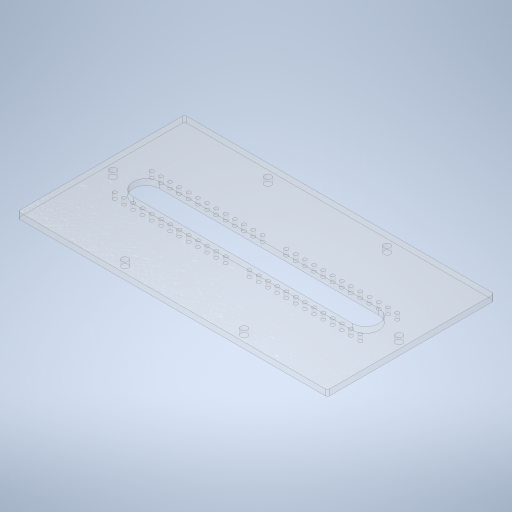
# Autodesk Inventor part: BT001_trajan20_21
Saved by Autodesk Inventor 2023 (Build 270158000, 158)
## iProperties
Company: HTBLA Kaindorf
RuleStatus: InUse
Created: 2022-08-03
Part Number: BT001_trajan20_21
Project: Zeichenmaschine_v2
Material: Acryl
Description: Platte Stepper Motoren
Document SubType Name: Modeling
Designer: trajan20
Density: 1.188 g/cm^3
Appearance: Transparent - farblos
Mass: 210.497 g
Surface Area: 764.437 cm^2
Volume: 177.186 cm^3
AfterDocNew0: iProperties-Editor_aufrufen
Author: jan
Keywords: 2021
Autodesk Inventor part; units mm, degrees
ref_plane "YZ Plane" through (0, 0, 0) normal (1, 0, 0) x (0, 1, 0)
ref_plane "XZ Plane" through (0, 0, 0) normal (0, 1, 0) x (-1, 0, 0)
ref_plane "XY Plane" through (0, 0, 0) normal (0, 0, 1) x (1, 0, 0)
derived "BT000_trajan20_22_Zeichenmaschine_neu_Masterskizze.ipt"
sketch "Skizze3" plane through (0, 0, 0) normal (0, 0, 1) x (1, 0, 0)
  line L0 (0, 0) -> (-140, 0)
  line L1 (-140, 0) -> (-140, 130)
  line L2 (-140, 260) -> (0, 260)
  line L3 (0, 260) -> (0, 0)
  line L4 (-140, 130) -> (-140, 260)
  line L5 (-70, 38) -> (-70, 222) construction
  line L6 (-81, 38) -> (-81, 222)
  line L7 (-59, 222) -> (-59, 38)
  arc A0 (-81, 38) -> (-59, 38) centre (-70, 38) ccw
  arc A1 (-59, 222) -> (-81, 222) centre (-70, 222) ccw
  circle A2 centre (-85.5, 27) radius 1.55
  circle A3 centre (-85.5, 58) radius 1.55
  circle A4 centre (-85.5, 34.75) radius 1.55
  circle A5 centre (-85.5, 42.5) radius 1.55
  line L8 (-85.5, 27) -> (-85.5, 242) construction
  circle A6 centre (-85.5, 50.25) radius 1.55
  line L9 (-88, 61.875) -> (-83, 61.875) construction
  circle A7 centre (-85.5, 96.75) radius 1.55
  circle A8 centre (-85.5, 89) radius 1.55
  circle A9 centre (-85.5, 81.25) radius 1.55
  circle A10 centre (-85.5, 73.5) radius 1.55
  circle A11 centre (-85.5, 65.75) radius 1.55
  line L10 (-88, 100.625) -> (-83, 100.625) construction
  circle A12 centre (-85.5, 112.25) radius 1.55
  circle A13 centre (-85.5, 120) radius 1.55
  circle A14 centre (-85.5, 104.5) radius 1.55
  line L11 (-70, 130) -> (-102, 130) construction
  circle A15 centre (-85.5, 225.25) radius 1.55
  circle A16 centre (-85.5, 217.5) radius 1.55
  circle A17 centre (-85.5, 209.75) radius 1.55
  circle A18 centre (-85.5, 202) radius 1.55
  circle A19 centre (-85.5, 194.25) radius 1.55
  circle A20 centre (-85.5, 186.5) radius 1.55
  circle A21 centre (-85.5, 178.75) radius 1.55
  circle A22 centre (-85.5, 171) radius 1.55
  circle A23 centre (-85.5, 163.25) radius 1.55
  circle A24 centre (-85.5, 155.5) radius 1.55
  circle A25 centre (-85.5, 147.75) radius 1.55
  circle A26 centre (-85.5, 140) radius 1.55
  circle A27 centre (-54.5, 27) radius 1.55
  circle A28 centre (-54.5, 34.75) radius 1.55
  circle A29 centre (-54.5, 42.5) radius 1.55
  circle A30 centre (-54.5, 50.25) radius 1.55
  circle A31 centre (-54.5, 58) radius 1.55
  circle A32 centre (-54.5, 65.75) radius 1.55
  circle A33 centre (-54.5, 73.5) radius 1.55
  circle A34 centre (-54.5, 81.25) radius 1.55
  circle A35 centre (-54.5, 89) radius 1.55
  circle A36 centre (-54.5, 96.75) radius 1.55
  circle A37 centre (-54.5, 104.5) radius 1.55
  circle A38 centre (-54.5, 112.25) radius 1.55
  circle A39 centre (-54.5, 120) radius 1.55
  circle A40 centre (-54.5, 140) radius 1.55
  circle A41 centre (-54.5, 147.75) radius 1.55
  circle A42 centre (-54.5, 155.5) radius 1.55
  circle A43 centre (-54.5, 163.25) radius 1.55
  circle A44 centre (-54.5, 171) radius 1.55
  circle A45 centre (-54.5, 178.75) radius 1.55
  circle A46 centre (-54.5, 186.5) radius 1.55
  circle A47 centre (-54.5, 194.25) radius 1.55
  circle A48 centre (-54.5, 202) radius 1.55
  circle A49 centre (-54.5, 209.75) radius 1.55
  circle A50 centre (-54.5, 217.5) radius 1.55
  circle A51 centre (-54.5, 225.25) radius 1.55
  circle A52 centre (-85.5, 233) radius 1.55
  circle A53 centre (-54.5, 233) radius 1.55
  point P0 (-85.5, 44.5)
  point P1 (-85.5, 75.5)
  point P2 (-54.5, 75.5)
  point P3 (-54.5, 44.5)
  point P4 (-70, 0)
  point P5 (-70, 10)
  point P6 (-130, 80)
  point P7 (-10, 80)
  point P8 (-102, 80)
  point P9 (-38, 80)
  point P10 (-70, 27)
  point P11 (-85.5, 61.875)
  point P12 (-85.5, 100.625)
  dimension "d4" = 260
  dimension "d5" = 140
  dimension "d22" = 10
  dimension "d23" = 10
  dimension "d26" = 10
  dimension "d57" = 80
  dimension "d60" = 184
  dimension "d61" = 11
  dimension "d62" = 11
  dimension "d63" = 3.1
  dimension "d64" = 31
  dimension "d65" = 3.1
  dimension "d66" = 3.1
  dimension "d67" = 7.75
  dimension "d68" = 3.1
  dimension "d70" = 15.5
  dimension "d71" = 7.75
  dimension "d72" = 3.1
  dimension "d73" = 7.75
  dimension "d74" = 5
  dimension "d75" = 3.875
  dimension "d76" = 5
  dimension "d77" = 11.625
  dimension "d78" = 32
  dimension "d85" = 38
  dimension "d86" = 70
  constraints: 54 centre point, 47 symmetric about line, 26 end point, 6 point on line, 5 parallel, 5 point on circle, 4 midpoint, 4 perpendicular, 4 tangent, 2 horizontal, 2 horizontal alignment, 1 vertical, 1 vertical alignment, 47 other
  measures "d4" distance between parallel lines of L2 L0
  measures "d5" distance between parallel lines of L1 L3
  measures "d22" distance from line of L0 point (-70, 10)
  measures "d23" distance from line of point (-10, 80) L3
  measures "d26" distance from line of L1 point (-130, 80)
  measures "d57" distance from line of L0 point (-130, 80)
  measures "d60" distance of L5.end L5.start
  measures "d61" radius of A0
  measures "d62" vertical distance of L8.start L5.start
  measures "d63" diameter of A2
  measures "d64" distance of A3.centre L8.start
  measures "d65" diameter of A3
  measures "d66" diameter of A4
  measures "d67" distance of L8.start A4.centre
  measures "d68" diameter of A5
  measures "d70" distance between parallel lines of L8 L5
  measures "d71" distance of A4.centre A5.centre
  measures "d72" diameter of A6
  measures "d73" distance of A6.centre A5.centre
  measures "d74" distance of L9.start L9.end
  measures "d75" distance from line of A3.centre L9
  measures "d76" distance of L10.start L10.end
  measures "d77" distance from line of A8.centre L10
  measures "d78" distance of L11.start L11.end
  measures "d85" distance from line of L0 L5.start
  measures "d86" distance from line of L3 L5.start
extrude "Extrusion3" add sketch "Skizze3" against normal blind 5 contours L0 L1 L4 L2 L3 | L6 A1 L7 A0 | A2 | A3 | A4 | A5 | A6 | A7 | A8 | A9 | A10 | A11 | A12 | A13 | A14 | A15 | A16 | A17 | A18 | A19 | A20 | A21 | A22 | A23 | A24 | A25 | A26 | A27 | A28 | A29 | A30 | A31 | A32 | A33 | A34 | A35 | A36 | A37 | A38 | A39 | A40 | A41 | A42 | A43 | A44 | A45 | A46 | A47 | A48 | A49 | A50 | A51 | A52 | A53
fillet "Rundung1" radius 2 4 edges at (0, 0, -2.5) (0, 260, -2.5) (-140, 260, -2.5) (-140, 0, -2.5)
hole "Bohrung1" at (-70, 10, 0) at (-130, 80, 0) at (-10, 80, 0) direction (0, 0, -1) diameter 5.5 end through all
ref_plane "Arbeitsebene3" through (0, 130, 0) normal (0, 1, 0) x (-1, 0, 0)
mirror "Spiegeln2" about plane through (0, 130, 0) normal (0, 1, 0) of "Bohrung1"
extrude "Extrusion7" cut sketch "Skizze3" against normal blind 20 contours L6 A1 L7 A0 | A2 | A3 | A4 | A5 | A6 | A7 | A8 | A9 | A10 | A11 | A12 | A13 | A14 | A15 | A16 | A17 | A18 | A19 | A20 | A21 | A22 | A23 | A24 | A25 | A26 | A27 | A28 | A29 | A30 | A31 | A32 | A33 | A34 | A35 | A36 | A37 | A38 | A39 | A40 | A41 | A42 | A43 | A44 | A45 | A46 | A47 | A48 | A49 | A50 | A51 | A52 | A53
equation "\"d23\" = d22"
equation "\"d26\" = d25"
equation "\"d25\" = d22"
